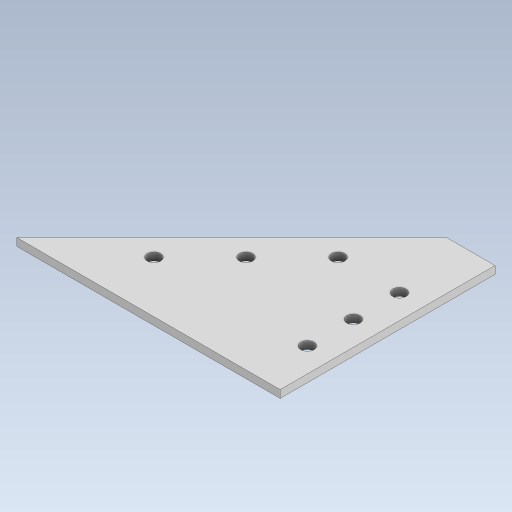
# Autodesk Inventor part: CH-1-01-FrontKneeJoint
Saved by Autodesk Inventor 2023 (Build 270158000, 158)
## iProperties
Created: 2023-02-06
Part Number: CH-1-01-FrontKneeJoint
Material: Generic
Document SubType Name: Modeling
Designer: Dave
Density: 1 g/cm^3
Appearance: Default
Author: Dave
Autodesk Inventor part; units mm, degrees
ref_plane "YZ Plane" through (0, 0, 0) normal (1, 0, 0) x (0, 1, 0)
ref_plane "XZ Plane" through (0, 0, 0) normal (0, 1, 0) x (-1, 0, 0)
ref_plane "XY Plane" through (0, 0, 0) normal (0, 0, 1) x (1, 0, 0)
sketch "Sketch1" plane through (0, 0, 0) normal (0, 1, 0) x (-1, 0, 0)
  line L0 (0, 0) -> (-101.6, 0) construction
  line L1 (-101.6, 0) -> (-101.6, -101.6) construction
  line L2 (-101.6, -101.6) -> (0, -101.6) construction
  line L3 (0, -101.6) -> (0, 0) construction
  line L4 (-101.6, 15.5049) -> (-81.6, 15.5049) construction
  line L5 (-81.6, 15.5049) -> (-81.6, -123.9701) construction
  line L6 (-81.6, -123.9701) -> (-101.6, -123.9701) construction
  line L7 (-101.6, -123.9701) -> (-101.6, 15.5049) construction
  line L8 (-81.6, -101.6) -> (54.3539, 34.3539) construction
  line L9 (54.3539, 34.3539) -> (40.2117, 48.496) construction
  line L10 (40.2117, 48.496) -> (-81.6, -73.3157) construction
  line L11 (-101.6, -101.6) -> (-81.6, -101.6)
  line L12 (-81.6, -101.6) -> (-3.5401, -23.5401)
  line L13 (-8.0303, -12.7) -> (-101.6, -12.7)
  line L14 (-101.6, -12.7) -> (-101.6, -101.6)
  circle A0 centre (-66.2, -72.0579) radius 5.1211
  circle A1 centre (-28.1, -33.9579) radius 5.1211
  circle A2 centre (-91.6, -33.9579) radius 5.1211
  circle A3 centre (-91.6, -72.0579) radius 5.1211
  line L15 (-81.6, -101.6) -> (-101.6, -121.6)
  line L16 (-101.6, -101.6) -> (-101.6, -121.6)
  line L17 (-28.1, -33.9579) -> (-66.2, -72.0579) construction
  line L18 (-8.0303, -12.7) -> (7.3, -12.7)
  line L19 (-3.5401, -23.5401) -> (7.3, -12.7)
  circle A4 centre (-47.15, -53.0079) radius 3.9521
  circle A5 centre (-91.6, -53.0079) radius 2.8637
  dimension "d0" = 101.6
  dimension "d1" = 101.6
  dimension "d2" = 20
  dimension "d3" = 20
  dimension "d4" = 45
  dimension "d11" = 10
  dimension "d13" = 10
  dimension "d15" = 25.4
  dimension "d16" = 38.1
  dimension "d17" = 88.9
  constraints: 40 end point, 9 point on line, 6 centre point, 5 parallel, 5 perpendicular, 4 horizontal, 3 collinear, 3 equal radius, 2 coincident, 2 horizontal alignment, 1 midpoint, 1 vertical, 1 vertical alignment
  measures "d0" distance of L2.end L1.end
  measures "d1" distance of L1.end L0.end
  measures "d2" distance of L5.end L6.end
  measures "d3" distance between parallel lines of L8 L10
  measures "d4" angle of L10 L5
  measures "d11" distance from line of L7 A2.centre
  measures "d13" distance between parallel lines of L8 L17
  measures "d15" distance of A0.centre A3.centre
  measures "d16" distance of A2.centre A3.centre
  measures "d17" distance between parallel lines of L13 L11
extrude "Extrusion1" add sketch "Sketch1" along normal blind 3.175 contours L14 L13 L18 L19 L12 L11 | A0 | A1 | A2 | A3 | A4 | A5
hole "Hole1" at (91.6, 0, -33.9579) at (91.6, 0, -72.0579) at (66.2, 0, -72.0579) at (28.1, 0, -33.9579) at (47.15, 0, -53.0079) at (91.6, 0, -53.0079) direction (0, 1, 0) diameter 5.5118 end through all clearance for "Flat Head Machine Screw" size "M5" standard "Ansi Metric M Profile"
equation "\"d3\" = d2"
body "Solid1"
